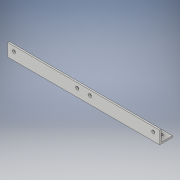
# Autodesk Inventor part: Middle short L
Saved by Autodesk Inventor 2017 (Build 210142000, 142)
## iProperties
Created: 2018-08-22
Part Number: Middle short L
Material: Generic
Document SubType Name: Modeling
Designer: sinner
Density: 1 g/cm^3
Appearance: Default
Author: sinner
Autodesk Inventor part; units mm, degrees
ref_plane "YZ Plane" through (0, 0, 0) normal (1, 0, 0) x (0, 1, 0)
ref_plane "XZ Plane" through (0, 0, 0) normal (0, 1, 0) x (-1, 0, 0)
ref_plane "XY Plane" through (0, 0, 0) normal (0, 0, 1) x (1, 0, 0)
sketch "Sketch1" plane through (0, 0, 0) normal (1, 0, 0) x (0, 1, 0)
  line L0 (0, 0) -> (25.4, 0)
  line L1 (3.2512, -25.4) -> (0, -25.4)
  line L2 (0, -25.4) -> (0, 0)
  line L3 (3.2512, -3.2512) -> (25.4, -3.2512)
  line L4 (3.2512, -25.4) -> (3.2512, -3.2512)
  line L5 (25.4, 0) -> (25.4, -3.2512)
  dimension "d0" = 25.4
  dimension "d1" = 3.2512
  constraints: 14 end point, 3 perpendicular, 2 horizontal, 2 parallel
  measures "d0" distance of L1.end L0.start
  measures "d1" distance of L1.start L1.end
extrude "Extrusion1" add sketch "Sketch1" along normal blind 304.8
sketch "Sketch2" plane through (0, 0, -25.4) normal (0, -1, 0) x (1, 0, 0)
  line L0 (0, 9.4488) -> (110.0411, 9.4488) construction
  line L1 (0, 25.4) -> (304.8, 25.4) projected
  circle A0 centre (12.7, 9.4488) radius 3.175
  circle A1 centre (139.7, 9.4488) radius 3.175
  line L2 (0, 0) -> (0, 25.4) projected
  line L3 (0, 0) -> (304.8, 0) projected
  line L4 (152.4, 25.4) -> (152.4, 0)
  circle A2 centre (292.1, 9.4488) radius 3.175
  circle A3 centre (165.1, 9.4488) radius 3.175
  dimension "d4" = 15.9512
  dimension "d5" = 6.35
  dimension "d6" = 12.7
  dimension "d7" = 139.7
  constraints: 4 centre point, 4 end point, 2 midpoint, 2 point on line, 2 symmetric about line, 1 equal radius, 1 horizontal, 2 other
  measures "d4" distance between parallel lines of L1 L0
  measures "d5" diameter of A1
  measures "d6" distance from line of L2 A0.centre
  measures "d7" distance from line of L2 A1.centre
extrude "Extrusion2" cut sketch "Sketch2" against normal blind 304.8 contours A0 | A1 | A2 | A3
sketch "Sketch3" plane through (0, 0, 0) normal (0, 0, 1) x (1, 0, 0)
  line L0 (0, 0) -> (0, 25.4) projected
  line L1 (0, 15.9512) -> (148.4119, 15.9512) construction
  line L2 (0, 0) -> (304.8, 0) projected
  circle A0 centre (12.7, 15.9512) radius 3.175
  circle A1 centre (139.7, 15.9512) radius 3.175
  line L3 (152.4, 0) -> (152.4, 21.95) construction
  circle A2 centre (292.1, 15.9512) radius 3.175
  circle A3 centre (165.1, 15.9512) radius 3.175
  dimension "d10" = 15.9512
  dimension "d11" = 6.35
  dimension "d12" = 12.7
  dimension "d13" = 139.7
  constraints: 4 centre point, 4 end point, 3 point on line, 2 symmetric about line, 1 equal radius, 1 horizontal, 1 midpoint, 1 vertical, 2 other
  measures "d10" distance between parallel lines of L2 L1
  measures "d11" diameter of A1
  measures "d12" distance from line of L0 A0.centre
  measures "d13" distance from line of L0 A1.centre
extrude "Extrusion3" cut sketch "Sketch3" against normal blind 304.8
body "Solid1"
